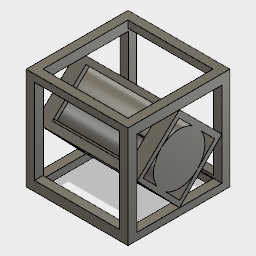
subtractive v1 (Autodesk Fusion 360 design; units mm, degrees)
Autodesk Fusion 360 part; units mm, degrees
sketch "Sketch1" plane through (0, 0, 0) normal (0, 1, 0) x (1, 0, 0)
  line L0 (-38.1, 38.1) -> (38.1, 38.1)
  line L1 (38.1, 38.1) -> (38.1, -38.1)
  line L2 (38.1, -38.1) -> (-38.1, -38.1)
  line L3 (-38.1, -38.1) -> (-38.1, 38.1)
  line L4 (-38.1, 38.1) -> (38.1, -38.1) construction
  line L5 (38.1, 38.1) -> (-38.1, -38.1) construction
  dimension "d1" = 76.2
  dimension "d2" = 76.2
  measures "d1" distance of L0.start L2.end
  measures "d2" distance of L1.end L2.end
extrude "Extrude1" add sketch "Sketch1" along normal blind 76.2 makes body 1
sketch "Sketch2" plane through (0, 76.2, 0) normal (0, 1, 0) x (-1, 0, 0)
  line L0 (38.1, 38.1) -> (-38.1, 38.1)
  line L1 (-38.1, 38.1) -> (-38.1, -38.1)
  line L2 (-38.1, -38.1) -> (38.1, -38.1)
  line L3 (38.1, -38.1) -> (38.1, 38.1)
  line L4 (31.75, -31.75) -> (-31.75, -31.75)
  line L5 (-31.75, -31.75) -> (-31.75, 31.75)
  line L6 (-31.75, 31.75) -> (31.75, 31.75)
  line L7 (31.75, 31.75) -> (31.75, -31.75)
  line L8 (31.75, -31.75) -> (-31.75, 31.75) construction
  line L9 (-31.75, -31.75) -> (31.75, 31.75) construction
  dimension "d5" = 63.5
  dimension "d6" = 63.5
  measures "d5" distance of L4.start L6.end
  measures "d6" distance of L4.start L4.end
extrude "Extrude2" cut sketch "Sketch2" against normal blind 81.28 contours L4 L5 L6 L7 bodies 1
sketch "Sketch3" plane through (0, 0, 38.1) normal (0, 0, 1) x (1, 0, 0)
  line L0 (-38.1, 0) -> (38.1, 0)
  line L1 (38.1, 0) -> (38.1, 76.2)
  line L2 (38.1, 76.2) -> (-38.1, 76.2)
  line L3 (-38.1, 76.2) -> (-38.1, 0)
  line L4 (-31.75, 70.8385) -> (31.75, 70.8385)
  line L5 (31.75, 70.8385) -> (31.75, 7.3385)
  line L6 (31.75, 7.3385) -> (-31.75, 7.3385)
  line L7 (-31.75, 7.3385) -> (-31.75, 70.8385)
  line L8 (-31.75, 70.8385) -> (31.75, 7.3385) construction
  line L9 (31.75, 70.8385) -> (-31.75, 7.3385) construction
  line L10 (-31.75, 76.2) -> (-31.75, 0)
  point P0 (0, 39.0885)
  dimension "d9" = 63.5
  dimension "d10" = 63.5
  measures "d9" distance of L4.start L6.end
  measures "d10" distance of L4.start L4.end
extrude "Extrude3" cut sketch "Sketch3" against normal blind 78.74 contours L4 L5 L6 L7 L10 bodies 1
sketch "Sketch4" plane through (38.1, 0, 0) normal (1, 0, 0) x (0, 0, -1)
  line L0 (-38.1, 0) -> (38.1, 0)
  line L1 (38.1, 0) -> (38.1, 76.2)
  line L2 (38.1, 76.2) -> (-38.1, 76.2)
  line L3 (-38.1, 76.2) -> (-38.1, 0)
  line L4 (-31.3693, 68.8615) -> (32.1307, 68.8615)
  line L5 (32.1307, 68.8615) -> (32.1307, 5.3615)
  line L6 (32.1307, 5.3615) -> (-31.3693, 5.3615)
  line L7 (-31.3693, 5.3615) -> (-31.3693, 68.8615)
  line L8 (-31.3693, 68.8615) -> (32.1307, 5.3615) construction
  line L9 (32.1307, 68.8615) -> (-31.3693, 5.3615) construction
  point P0 (0.3807, 37.1115)
  dimension "d13" = 63.5
  dimension "d14" = 63.5
  measures "d13" distance of L4.start L6.end
  measures "d14" distance of L4.start L4.end
extrude "Extrude4" cut sketch "Sketch4" against normal blind 81.28 contours L4 L5 L6 L7 bodies 1
sketch "Sketch5" plane through (0, 0, 0) normal (1, 0, 0) x (0, 0, -1)
sketch "Sketch6" plane through (38.1, 0, 0) normal (1, 0, 0) x (0, 0, -1)
  line L0 (32.1307, 68.8615) -> (32.1307, 5.3615)
  line L1 (32.1307, 5.3615) -> (-31.3693, 5.3615)
  line L2 (-31.3693, 5.3615) -> (-31.3693, 68.8615)
  line L3 (-31.3693, 68.8615) -> (32.1307, 68.8615)
  line L4 (-38.1, 0) -> (38.1, 0)
  line L5 (38.1, 0) -> (38.1, 76.2)
  line L6 (38.1, 76.2) -> (-38.1, 76.2)
  line L7 (-38.1, 76.2) -> (-38.1, 0)
  line L8 (0.3807, 68.8615) -> (-31.3693, 38.4696)
  line L9 (-31.3693, 38.4696) -> (0.3807, 5.3615)
  line L10 (0.3807, 5.3615) -> (32.1307, 37.1115)
  line L11 (32.1307, 37.1115) -> (0.3807, 68.8615)
  point P0 (0.5787, 32.6023)
  point P1 (0.5786, 31.857)
extrude "Extrude5" add sketch "Sketch6" against normal blind 76.2 separate body contours L8 L9 L10 L11 makes body 2
sketch "Sketch7" plane through (-38.1, 0, 0) normal (-1, 0, 0) x (0, 0, 1)
  line L0 (-0.3807, 68.8615) -> (-32.1307, 37.1115)
  line L1 (-32.1307, 37.1115) -> (-0.3807, 5.3615)
  line L2 (-0.3807, 5.3615) -> (31.3693, 38.4696)
  line L3 (31.3693, 38.4696) -> (-0.3807, 68.8615)
  line L4 (0, 63.5) -> (26.67, 38.1)
  line L5 (0, 63.5) -> (-26.67, 36.83)
  line L6 (-26.67, 36.83) -> (-0.5866, 10.0345)
  line L7 (26.67, 38.1) -> (-0.5866, 10.0345)
extrude "Extrude6" cut sketch "Sketch7" against normal blind 76.2 contours L4 L5 L6 L7 bodies 2
sketch "Sketch8" plane through (0, 2.7587, -2.8767) normal (0, -0.692149, 0.721755) x (1, 0, 0)
  line L0 (38.1, 3.6062) -> (38.1, 49.4778)
  line L1 (38.1, 49.4778) -> (-38.1, 49.4778)
  line L2 (-38.1, 49.4778) -> (-38.1, 3.6062)
  line L3 (-38.1, 3.6062) -> (38.1, 3.6062)
  line L4 (-25.4, 45.72) -> (-25.4, 10.16)
  line L5 (-25.4, 10.16) -> (27.94, 10.16)
  line L6 (27.94, 10.16) -> (27.94, 45.72)
  line L7 (27.94, 45.72) -> (-25.4, 45.72)
extrude "Extrude7" cut sketch "Sketch8" against normal blind 45.72 contours L4 L5 L6 L7 bodies 2
sketch "Sketch9" plane through (0, 2.4904, 2.4904) normal (0, -0.707107, -0.707107) x (-1, 0, 0)
  line L0 (-38.1, 48.9616) -> (-38.1, 4.0604)
  line L1 (-38.1, 4.0604) -> (38.1, 4.0604)
  line L2 (38.1, 4.0604) -> (38.1, 48.9616)
  line L3 (38.1, 48.9616) -> (-38.1, 48.9616)
  line L4 (-27.94, 10.16) -> (28.8286, 10.16)
  line L5 (28.8286, 10.16) -> (28.8286, 44.9013)
  line L6 (28.8286, 44.9013) -> (-27.94, 44.9013)
  line L7 (-27.94, 44.9013) -> (-27.94, 10.16)
extrude "Extrude8" cut sketch "Sketch9" against normal blind 45.72 contours L4 L5 L6 L7 bodies 2
sketch "Sketch10" plane through (38.1, 0, 0) normal (1, 0, 0) x (0, 0, -1)
  line L0 (26.67, 36.83) -> (0.5866, 10.0345)
  line L1 (0.5866, 10.0345) -> (-26.67, 38.1)
  line L2 (-26.67, 38.1) -> (0, 63.5)
  line L3 (0, 63.5) -> (26.67, 36.83)
  line L4 (32.1307, 37.1115) -> (0.3807, 68.8615)
  line L5 (0.3807, 68.8615) -> (-31.3693, 38.4696)
  line L6 (-31.3693, 38.4696) -> (0.3807, 5.3615)
  line L7 (0.3807, 5.3615) -> (32.1307, 37.1115)
  circle A0 centre (0.1467, 37.1161) radius 19.2095
extrude "Extrude9" add sketch "Sketch10" against normal blind 73.66 contours L0 L1 L2 L3 A0 bodies 2
extrude "Extrude10" add 1 faces at (-35.56, 41.068, -3.9719) along direction (-1, 0, 0) blind 2.54 on bodies 2 bodies 2
